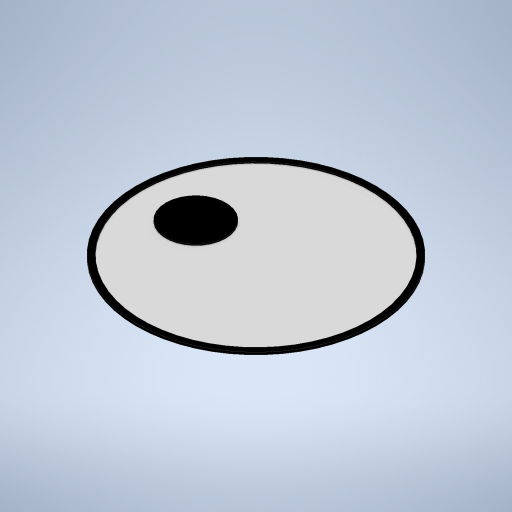
# Autodesk Inventor part: oko
Saved by Autodesk Inventor 2023 (Build 270158000, 158)
## iProperties
Created: 2023-07-08
Part Number: oko
Material: Ogólny
Document SubType Name: Modeling
Designer: Kamil
Density: 1 g/cm^3
Appearance: Domyślna
Author: Kamil
Autodesk Inventor part; units mm, degrees
ref_plane "YZ Plane" through (0, 0, 0) normal (1, 0, 0) x (0, 1, 0)
ref_plane "XZ Plane" through (0, 0, 0) normal (0, 1, 0) x (-1, 0, 0)
ref_plane "XY Plane" through (0, 0, 0) normal (0, 0, 1) x (1, 0, 0)
sketch "Szkic1" plane through (0, 0, 0) normal (0, 1, 0) x (-1, 0, 0)
  circle A0 centre (0, 0) radius 10
  dimension "d0" = 20
  constraints: 1 centre point, 1 coincident
  measures "d0" diameter of A0
extrude "Wyciągnięcie proste1" add sketch "Szkic1" along normal blind 0.1
sketch "Szkic2" plane through (0, 0.1, 0) normal (0, 1, 0) x (1, 0, 0)
  circle A0 centre (0, 0) radius 10 projected
  circle A1 centre (0, 0) radius 9.5
  circle A2 centre (-5.0365, 0) radius 2.5
  dimension "d3" = 19
  dimension "d6" = 5
  constraints: 2 centre point, 1 coincident
  measures "d3" diameter of A1
  measures "d6" diameter of A2
extrude "Wyciągnięcie proste2" add sketch "Szkic2" along normal blind 0.1
